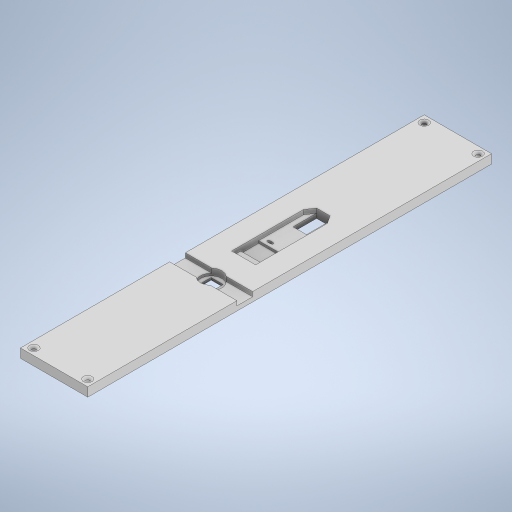
# Autodesk Inventor part: BackboardV3
Saved by Autodesk Inventor 2024 (Build 280153000, 153)
## iProperties
Created: 2024-03-08
Part Number: BackboardV3
Material: Všeobecné
Document SubType Name: Modeling
Designer: zak
Density: 1 g/cm^3
Appearance: Výchozí
Author: zak
Autodesk Inventor part; units mm, degrees
ref_plane "YZ Plane" through (0, 0, 0) normal (1, 0, 0) x (0, 1, 0)
ref_plane "XZ Plane" through (0, 0, 0) normal (0, 1, 0) x (-1, 0, 0)
ref_plane "XY Plane" through (0, 0, 0) normal (0, 0, 1) x (1, 0, 0)
sketch "Náčrt1" plane through (0, 0, 0) normal (0, 1, 0) x (-1, 0, 0)
  line L0 (0, 0) -> (-30, 0)
  line L1 (-30, 0) -> (-30, -180)
  line L2 (-30, -180) -> (0, -180)
  line L3 (0, -180) -> (0, 0)
  dimension "d0" = 30
  dimension "d1" = 180
  constraints: 8 end point, 2 parallel, 1 horizontal, 1 perpendicular
  measures "d0" distance of L2.end L1.end
  measures "d1" distance of L1.end L0.end
extrude "Vysunutí1" add sketch "Náčrt1" along normal blind 4
sketch "Náčrt2" plane through (0, 4, 0) normal (0, 1, 0) x (1, 0, 0)
  line L0 (30, 0) -> (30, 180) projected
  line L1 (30, 180) -> (0, 180) projected
  line L2 (0, 180) -> (0, 0) projected
  line L3 (0, 0) -> (30, 0) projected
  line L4 (15, 0) -> (15, 180) construction
  line L5 (9.65, 84.5) -> (20.35, 84.5)
  line L6 (20.35, 84.5) -> (20.35, 120)
  line L7 (20.35, 120) -> (9.65, 120)
  line L8 (9.65, 120) -> (9.65, 84.5)
  line L9 (12, 109.5) -> (18, 109.5)
  line L10 (18, 109.5) -> (18, 120)
  line L11 (18, 120) -> (12, 120)
  line L12 (12, 120) -> (12, 109.5)
  line L13 (18, 120) -> (20.35, 116.5)
  line L14 (12, 120) -> (9.65, 116.5)
  dimension "d4" = 10.7
  dimension "d5" = 35.5
  dimension "d6" = 60
  dimension "d7" = 6
  dimension "d8" = 10.5
  dimension "d9" = 32
  constraints: 22 end point, 4 parallel, 2 horizontal, 2 midpoint, 2 perpendicular, 1 collinear, 1 point on line, 1 symmetric about line, 2 other
  measures "d4" distance of L7.end L6.end
  measures "d5" distance of L5.end L6.end
  measures "d6" distance between parallel lines of L1 L7
  measures "d7" distance of L11.end L10.end
  measures "d8" distance of L10.end L9.end
  measures "d9" distance from line of L5 L13.end
extrude "Vysunutí2" cut sketch "Náčrt2" against normal blind 2 contours L8 L14 L12 L9 L10 L13 L6 L5
extrude "Vysunutí3" cut sketch "Náčrt2" against normal blind 4 contours L7 L10 L9 L12
sketch "Náčrt3" plane through (0, 4, 0) normal (0, 1, 0) x (1, 0, 0)
  circle A0 centre (15, 70) radius 4.75
  line L0 (30, 0) -> (30, 180) projected
  line L1 (30, 180) -> (0, 180) projected
  line L2 (0, 180) -> (0, 0) projected
  line L3 (0, 0) -> (30, 0) projected
  line L4 (12, 120) -> (18, 120) projected
  line L5 (18, 120) -> (20.35, 116.5) projected
  line L6 (20.35, 116.5) -> (20.35, 84.5) projected
  line L7 (20.35, 84.5) -> (9.65, 84.5) projected
  line L8 (9.65, 84.5) -> (9.65, 116.5) projected
  line L9 (9.65, 116.5) -> (12, 120) projected
  line L10 (15, 0) -> (15, 180) construction
  line L11 (12.3, 67.3) -> (17.7, 67.3)
  line L12 (17.7, 67.3) -> (17.7, 72.7)
  line L13 (17.7, 72.7) -> (12.3, 72.7)
  line L14 (12.3, 72.7) -> (12.3, 67.3)
  line L15 (0, 66.5) -> (30, 66.5)
  line L16 (30, 66.5) -> (30, 73.5)
  line L17 (30, 73.5) -> (0, 73.5)
  line L18 (0, 73.5) -> (0, 66.5)
  point P0 (11.7887, 73.5)
  point P1 (11.7887, 66.5)
  point P2 (18.2113, 73.5)
  point P3 (18.2113, 66.5)
  dimension "d14" = 9.5
  dimension "d15" = 70
  dimension "d16" = 5.4
  dimension "d17" = 5.4
  dimension "d18" = 2.7
  dimension "d19" = 7
  dimension "d20" = 3.5
  constraints: 18 end point, 4 parallel, 3 point on line, 2 horizontal, 2 midpoint, 2 perpendicular, 1 centre point, 1 coincident, 1 other
  measures "d14" diameter of A0
  measures "d15" distance from line of L3 A0.centre
  measures "d16" distance of L11.end L12.end
  measures "d17" distance of L11.start L11.end
  measures "d18" distance from line of L13 point (15, 70)
  measures "d19" distance of L15.end L16.end
  measures "d20" distance from line of A0.centre L17
extrude "Vysunutí4" cut sketch "Náčrt3" against normal blind 2 contours A0 L17 L0 L15 | A0 L15 L2 L17
extrude "Vysunutí5" cut sketch "Náčrt3" against normal blind 3 contours A0 L15 L17 | L17 A0 | A0 L15
extrude "Vysunutí6" cut sketch "Náčrt3" against normal blind 4 contours L14 L13 L12 L11
sketch "Náčrt4" plane through (0, 2, 0) normal (0, 1, 0) x (1, 0, 0)
  line L0 (20.35, 116.5) -> (20.35, 84.5) construction
  line L1 (18, 120) -> (20.35, 116.5) construction
  line L2 (18, 109.5) -> (18, 120) construction
  line L3 (12, 109.5) -> (18, 109.5) construction
  line L4 (12, 120) -> (12, 109.5) construction
  line L5 (9.65, 116.5) -> (12, 120) construction
  line L6 (9.65, 84.5) -> (9.65, 116.5) construction
  line L7 (20.35, 84.5) -> (9.65, 84.5) construction
  line L8 (9.65, 88.5) -> (20.35, 88.5)
  line L9 (20.35, 88.5) -> (20.35, 96.5)
  line L10 (20.35, 96.5) -> (9.65, 96.5)
  line L11 (9.65, 96.5) -> (9.65, 88.5)
  ellipse E0 centre (12.85, 98.5) end of major axis (14.1807, 98.5) minor radius 0.6195
  point P0 (0, 0)
  dimension "d27" = 8
  dimension "d28" = 4
  dimension "d29" = 14
  dimension "d30" = 3.2
  constraints: 8 end point, 2 parallel, 2 point on line, 1 centre point, 1 horizontal, 1 perpendicular, 1 other
  measures "d27" distance between parallel lines of L10 L8
  measures "d28" distance between parallel lines of L7 L8
  measures "d29" distance from line of L7 E0.centre
  measures "d30" distance from line of L6 E0.centre
extrude "Vysunutí7" cut sketch "Náčrt4" against normal blind 4 contours E0
extrude "Vysunutí8" cut sketch "Náčrt4" against normal blind 1 contours L11 L10 L9 L8
sketch "Náčrt5" plane through (0, 4, 0) normal (0, 1, 0) x (1, 0, 0)
  line L0 (0, 0) -> (30, 0) projected
  line L1 (0, 66.5) -> (0, 0) projected
  line L2 (15, 0) -> (15, 180) construction
  line L3 (30, 180) -> (0, 180) construction
  line L4 (30, 0) -> (30, 180) construction
  line L5 (30, 90) -> (0, 90) construction
  point P0 (3, 3)
  point P1 (27, 3)
  point P2 (3, 177)
  point P3 (27, 177)
  dimension "d35" = 3
  dimension "d36" = 3
  constraints: 4 end point, 3 midpoint, 3 symmetric about line, 1 horizontal
  measures "d35" distance from line of L0 point (3, 3)
  measures "d36" distance from line of L1 point (3, 3)
hole "Díra1" at (3, 4, -3) at (27, 4, -3) at (3, 4, -177) at (27, 4, -177) direction (0, -1, 0) diameter 2 end through all
fillet "Zaoblení1" radius 1 4 edges at (27, 4, -4) (3, 4, -4) (27, 4, -178) (3, 4, -178)
equation "\"d18\" = 0.5 * d16"
equation "\"d20\" = 0.5 * d19"
